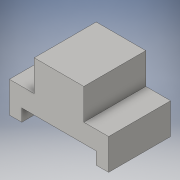
# Autodesk Inventor part: Figure 7_27_2
Saved by Autodesk Inventor 2016 (Build 200138000, 138)
## iProperties
Created: 2016-07-18
Part Number: Figure 7_27_2
Material: Generic
Document SubType Name: Modeling
Designer: cfkguest
Density: 1 g/cm^3
Appearance: Default
Author: cfkguest
Autodesk Inventor part; units mm, degrees
ref_plane "YZ Plane" through (0, 0, 0) normal (1, 0, 0) x (0, 1, 0)
ref_plane "XZ Plane" through (0, 0, 0) normal (0, 1, 0) x (-1, 0, 0)
ref_plane "XY Plane" through (0, 0, 0) normal (0, 0, 1) x (1, 0, 0)
sketch "Sketch1" plane through (0, 0, 0) normal (0, 0, 1) x (1, 0, 0)
  line L0 (-18.2958, -15.2546) -> (32.5042, -15.2546)
  line L1 (32.5042, -15.2546) -> (32.5042, 16.4954)
  line L2 (32.5042, 16.4954) -> (-18.2958, 16.4954)
  line L3 (-18.2958, 16.4954) -> (-18.2958, -15.2546)
  point P0 (0, 0)
  dimension "d0" = 50.8
  dimension "d1" = 31.75
  constraints: 8 end point, 2 parallel, 1 horizontal, 1 perpendicular
  measures "d0" distance of L1.end L2.end
  measures "d1" distance of L2.end L0.start
extrude "Extrusion1" add sketch "Sketch1" along normal blind 31.75
sketch "Sketch2" plane through (0, 0, 31.75) normal (0, 0, 1) x (1, 0, 0)
  line L0 (32.5042, 16.4954) -> (-18.2958, 16.4954) projected
  line L1 (32.5042, -15.2546) -> (32.5042, 16.4954) projected
  line L2 (19.8042, 16.4954) -> (32.5042, 16.4954)
  line L3 (32.5042, 16.4954) -> (32.5042, 0.6204)
  line L4 (32.5042, 0.6204) -> (19.8042, 0.6204)
  line L5 (19.8042, 0.6204) -> (19.8042, 16.4954)
  line L6 (-18.2958, 16.4954) -> (-18.2958, -15.2546) projected
  line L7 (-18.2958, 0.6204) -> (-5.5958, 0.6204)
  line L8 (-5.5958, 0.6204) -> (-5.5958, 16.4954)
  line L9 (-5.5958, 16.4954) -> (-18.2958, 16.4954)
  line L10 (-18.2958, 16.4954) -> (-18.2958, 0.6204)
  point P0 (0, 0)
  dimension "d4" = 15.875
  dimension "d5" = 12.7
  dimension "d6" = 15.875
  dimension "d7" = 12.7
  constraints: 16 end point, 4 parallel, 2 horizontal, 2 midpoint, 2 perpendicular, 2 point on line
  measures "d4" distance of L4.end L2.start
  measures "d5" distance of L3.end L4.end
  measures "d6" distance of L7.end L8.end
  measures "d7" distance of L7.start L7.end
extrude "Extrusion2" cut sketch "Sketch2" against normal blind 31.75
sketch "Sketch3" plane through (0, 0, 31.75) normal (0, 0, 1) x (1, 0, 0)
  line L0 (-18.2958, -15.2546) -> (32.5042, -15.2546) projected
  line L1 (-11.9458, -15.2546) -> (26.1542, -15.2546)
  line L2 (26.1542, -15.2546) -> (26.1542, -8.9046)
  line L3 (26.1542, -8.9046) -> (-11.9458, -8.9046)
  line L4 (-11.9458, -8.9046) -> (-11.9458, -15.2546)
  line L5 (-18.2958, 0.6204) -> (-18.2958, -15.2546) projected
  line L6 (32.5042, -15.2546) -> (32.5042, 0.6204) projected
  point P0 (0, 0)
  dimension "d10" = 6.35
  dimension "d11" = 6.35
  dimension "d12" = 6.35
  constraints: 8 end point, 2 parallel, 1 horizontal, 1 perpendicular, 1 point on line
  measures "d10" distance between parallel lines of L5 L4
  measures "d11" distance between parallel lines of L6 L2
  measures "d12" distance of L3.end L1.start
extrude "Extrusion3" cut sketch "Sketch3" against normal blind 31.75
body "Solid1"
